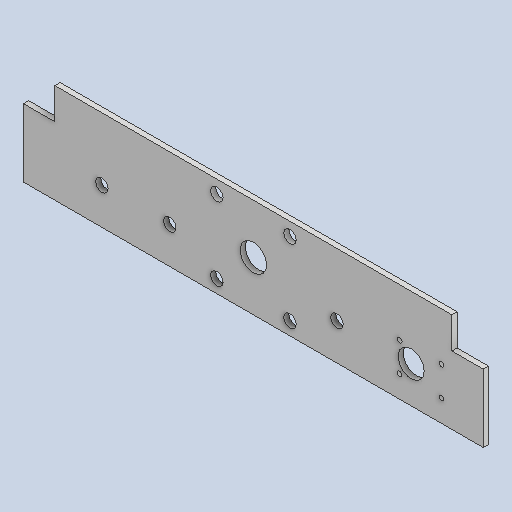
# Autodesk Inventor part: Suporte _ Motores
Saved by Autodesk Inventor 2026.2 (Build 302298010, 298A)
## iProperties
Created: 2026-02-20
Part Number: Suporte _ Motores
Material: Generic
Document SubType Name: Modeling
Designer: 062210040
Density: 1 g/cm^3
Appearance: Default
Author: 062210040
Autodesk Inventor part; units mm, degrees
ref_plane "YZ Plane" through (0, 0, 0) normal (1, 0, 0) x (0, 1, 0)
ref_plane "XZ Plane" through (0, 0, 0) normal (0, 1, 0) x (-1, 0, 0)
ref_plane "XY Plane" through (0, 0, 0) normal (0, 0, 1) x (1, 0, 0)
sketch "Sketch1" plane through (0, 0, 0) normal (0, 0, 1) x (1, 0, 0)
  line L0 (0, 0) -> (0, 65)
  line L1 (0, 65) -> (30, 65)
  line L2 (30, 65) -> (30, 95)
  line L3 (30, 95) -> (410, 95)
  line L4 (410, 95) -> (410, 65)
  line L5 (410, 65) -> (440, 65)
  line L6 (440, 65) -> (440, 0)
  line L7 (440, 0) -> (0, 0)
  circle A0 centre (220, 47.5) radius 12.7
  circle A1 centre (140, 35) radius 6
  line L8 (220, 146.6753) -> (220, -14.9007)
  circle A2 centre (371, 35) radius 12.5
  circle A3 centre (300, 35) radius 6
  circle A4 centre (400, 49) radius 2.25
  circle A5 centre (360, 49) radius 2.25
  circle A6 centre (400, 21) radius 2.25
  circle A7 centre (360, 21) radius 2.25
  circle A8 centre (75, 35) radius 6
  line L9 (0, 0) -> (0.2906, 0)
  point P0 (0.1453, 0)
  dimension "d1" = 65
  dimension "d2" = 30
  dimension "d3" = 30
  dimension "d4" = 380
  dimension "d5" = 30
  dimension "d6" = 30
  dimension "d7" = 25.4
  dimension "d18" = 12
  dimension "d21" = 140
  dimension "d37" = 0
  dimension "d39" = 190
  dimension "d40" = 35
  dimension "d45" = 12
  dimension "d46" = 35
  dimension "d47" = 75
  dimension "d49" = 11
  dimension "d50" = 11
  dimension "d51" = 14
  dimension "d52" = 14
  dimension "d53" = 29
  dimension "d55" = 29
  dimension "d56" = 28
  dimension "d57" = 71
  dimension "d58" = 0
  dimension "d61" = 25
  dimension "d62" = 4.5
  dimension "d63" = 4.5
  dimension "d64" = 4.5
  dimension "d65" = 4.5
  dimension "d67" = 0
  dimension "d68" = 14
  dimension "d85" = 47.5
  constraints: 20 end point, 9 centre point, 5 perpendicular, 4 horizontal, 3 vertical, 1 midpoint, 1 symmetric about line, 1 other
  measures "d1" distance of L0.start L0.end
  measures "d2" distance of L0.end L1.end
  measures "d3" distance of L1.end L2.end
  measures "d4" distance of L2.end L3.end
  measures "d5" distance of L3.end L4.end
  measures "d6" distance of L4.end L5.end
  measures "d7" diameter of A0
  measures "d18" diameter of A1
  measures "d21" distance from line of L0 A1.centre
  measures "d37" distance from line of A0.centre L8
  measures "d39" distance between parallel lines of L8 L4
  measures "d40" distance from line of L7 A1.centre
  measures "d45" diameter of A8
  measures "d46" distance from line of L7 A8.centre
  measures "d47" distance from line of L0 A8.centre
  measures "d49" horizontal distance of A5.centre A2.centre
  measures "d50" horizontal distance of A7.centre A2.centre
  measures "d51" vertical distance of A2.centre A7.centre
  measures "d52" vertical distance of A5.centre A2.centre
  measures "d53" horizontal distance of A2.centre A4.centre
  measures "d55" horizontal distance of A2.centre A6.centre
  measures "d56" distance of A4.centre A6.centre
  measures "d57" distance of A2.centre A3.centre
  measures "d58" distance from line of point (0.145, 0) L7
  measures "d61" diameter of A2
  measures "d62" diameter of A5
  measures "d63" diameter of A7
  measures "d64" diameter of A6
  measures "d65" diameter of A4
  measures "d67" vertical distance of A3.centre A2.centre
  measures "d68" vertical distance of A2.centre A4.centre
  measures "d85" distance from line of L7 A0.centre
extrude "Extrusion1" add sketch "Sketch1" along normal blind 5 contours L0 L1 L2 L3 L8 A0 L7 | L8 A0 L3 L4 L5 L6 L7
sketch "Sketch2" plane through (0, 0, 5) normal (0, 0, 1) x (1, 0, 0)
  circle A0 centre (185, 82.5) radius 6
  circle A1 centre (255, 82.5) radius 6
  circle A2 centre (185, 12.5) radius 6
  circle A3 centre (255, 12.5) radius 6
  circle A4 centre (220, 47.5) radius 12.7 projected
  point P0 (0, 0)
  dimension "d71" = 12
  dimension "d72" = 12
  dimension "d73" = 12
  dimension "d74" = 12
  dimension "d75" = 35
  dimension "d76" = 35
  dimension "d77" = 70
  dimension "d78" = 35
  dimension "d79" = 35
  dimension "d80" = 70
  dimension "d81" = 35
  dimension "d82" = 35
  constraints: 4 centre point
  measures "d71" diameter of A0
  measures "d72" diameter of A1
  measures "d73" diameter of A2
  measures "d74" diameter of A3
  measures "d75" horizontal distance of A4.centre A3.centre
  measures "d76" horizontal distance of A4.centre A2.centre
  measures "d77" distance of A2.centre A3.centre
  measures "d78" horizontal distance of A4.centre A0.centre
  measures "d79" horizontal distance of A4.centre A1.centre
  measures "d80" distance of A0.centre A1.centre
  measures "d81" horizontal distance of A4.centre A3.centre
  measures "d82" horizontal distance of A4.centre A0.centre
extrude "Extrusion2" cut sketch "Sketch2" against normal through all contours A0 | A1 | A2 | A3
body "Solid1"
